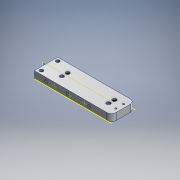
# Autodesk Inventor part: c-head-flange
Saved by Autodesk Inventor 2016 (Build 200138000, 138)
## iProperties
Created: 2015-05-12
Part Number: c-head-flange
Material: Aluminum 6061
Document SubType Name: Modeling
Designer: as
Mass: 12.4418 g
Surface Area: 45.4358 cm^2
Volume: 4.60808 cm^3
Density: 2.7 g/cm^3
Appearance: Aluminum - Flat
Author: as
Autodesk Inventor part; units mm, degrees
ref_plane "YZ Plane" through (0, 0, 0) normal (1, 0, 0) x (0, 1, 0)
ref_plane "XZ Plane" through (0, 0, 0) normal (0, 1, 0) x (-1, 0, 0)
ref_plane "XY Plane" through (0, 0, 0) normal (0, 0, 1) x (1, 0, 0)
sketch "Sketch1" plane through (0, 0, 0) normal (0, 0, 1) x (1, 0, 0)
  line L0 (-6, -20) -> (60, -20)
  line L1 (60, -20) -> (60, 0)
  line L2 (60, 0) -> (-6, 0)
  line L3 (-6, 0) -> (-6, -20)
  point P0 (0, 0)
  dimension "d2" = 20
  dimension "d3" = 66
  dimension "d8" = 60
  dimension "d9" = 0
  constraints: 8 end point, 2 parallel, 1 horizontal, 1 perpendicular
  measures "d2" distance of L0.end L1.end
  measures "d3" distance of L1.end L2.end
  measures "d8" distance from line of point (0, 0) L1
  measures "d9" distance from line of point (0, 0) L2
extrude "Extrusion1" add sketch "Sketch1" along normal blind 6
sketch "Sketch5" plane through (0, 0, 6) normal (0, 0, 1) x (1, 0, 0)
  line L0 (-6, 0) -> (-6, -20) projected
  point P0 (0, 0)
  point P1 (-3, -3)
  point P2 (-3, -17)
  dimension "d48" = 3
  dimension "d50" = 17
  dimension "d51" = 3
  dimension "d53" = 3
  measures "d48" horizontal distance of L0.start point (-3, -3)
  measures "d50" vertical distance of L0.start point (-3, -17)
  measures "d51" distance from line of L0 point (-3, -3)
  measures "d53" distance from line of L0 point (-3, -17)
hole "Hole6" at (-3, -3, 6) at (-3, -17, 6) direction (0, 0, -1) diameter 3 end through all
sketch "Sketch7" plane through (0, 0, 0) normal (0, 0, -1) x (-1, 0, 0)
  line L0 (-60, 0) -> (0, 0) projected
  line L1 (6, 0) -> (6, -20) projected
  point P0 (-57, -6.75)
  point P1 (-57, -13.25)
  dimension "d68" = 6.75
  dimension "d69" = 63
  dimension "d70" = 6.5
  dimension "d71" = 63
  measures "d68" distance from line of L0 point (-57, -6.75)
  measures "d69" distance from line of L1 point (-57, -6.75)
  measures "d70" distance of point (-57, -13.25) point (-57, -6.75)
  measures "d71" distance from line of point (-57, -13.25) L1
hole "Hole9" at (57, -13.25, 0) at (57, -6.75, 0) direction (0, 0, 1) diameter 1.567 end through all thread size "M2x0.4" class "6H" standard "ISO Metric profile"
sketch "Sketch8" plane through (0, 0, 0) normal (0, 0, -1) x (-1, 0, 0)
  line L0 (-51.7988, -18) -> (-47.7988, -18)
  line L1 (-47.7988, -2) -> (-51.7988, -2)
  line L2 (-53.7988, -4) -> (-53.7988, -16)
  line L3 (-53.7988, -18) -> (-45.7988, -2) construction
  line L4 (-45.7988, -18) -> (-53.7988, -2) construction
  arc A0 (-53.7988, -16) -> (-51.7988, -18) centre (-51.7988, -16) ccw
  arc A1 (-47.7988, -18) -> (-45.9448, -16.75) centre (-47.7988, -16) ccw
  arc A2 (-45.9448, -3.25) -> (-47.7988, -2) centre (-47.7988, -4) ccw
  arc A3 (-51.7988, -2) -> (-53.7988, -4) centre (-51.7988, -4) ccw
  line L5 (-44.0907, -15.5) -> (-1.7988, -15.5)
  line L6 (-1.7988, -4.5) -> (-44.0907, -4.5)
  line L7 (0.2012, -6.5) -> (0.2012, -13.5)
  arc A4 (-1.7988, -15.5) -> (0.2012, -13.5) centre (-1.7988, -13.5) ccw
  arc A5 (0.2012, -6.5) -> (-1.7988, -4.5) centre (-1.7988, -6.5) ccw
  arc A6 (-44.0907, -15.5) -> (-45.9448, -16.75) centre (-44.0907, -17.5) ccw
  arc A7 (-45.9448, -3.25) -> (-44.0907, -4.5) centre (-44.0907, -2.5) ccw
  line L8 (-60, 0) -> (6, 0) projected
  line L9 (6, -20) -> (-60, -20) projected
  point P0 (-49.7988, -10)
  point P1 (-45.7988, -16)
  point P2 (-45.8623, -4.5)
  point P3 (-44.7988, -15.5)
  dimension "d124" = 16
  dimension "d125" = 8
  dimension "d126" = 2
  dimension "d149" = 2
  dimension "d150" = 2
  dimension "d165" = 10
  dimension "d166" = 4.5
  dimension "d167" = 4.5
  dimension "d168" = 66
  dimension "d169" = 10
  dimension "d170" = 2
  dimension "d171" = 2
  dimension "d172" = 54
  dimension "d173" = 5.7988
  dimension "d174" = 4
  dimension "d175" = 45
  constraints: 18 point on circle, 16 end point, 16 tangent, 8 centre point, 8 point on line, 5 equal radius, 4 parallel, 2 midpoint, 1 horizontal, 1 vertical
  measures "d124" distance of L4.end L3.start
  measures "d125" distance of L3.start L4.start
  measures "d126" radius of A0
  measures "d149" radius of A4
  measures "d150" radius of A6
  measures "d165" distance from line of L8 point (-49.799, -10)
  measures "d166" distance between parallel lines of L8 L6
  measures "d167" distance between parallel lines of L9 L5
  measures "d168" distance of L8.start L8.end
  measures "d169" distance from line of point (-49.799, -10) L9
  measures "d170" distance between parallel lines of L8 L1
  measures "d171" distance between parallel lines of L9 L0
  measures "d172" distance between parallel lines of L7 L2
  measures "d173" distance from line of L8.end L7
  measures "d174" distance from line of point (-45.799, -16) L9
  measures "d175" distance from line of point (-44.799, -15.5) L7
extrude "Extrusion2" cut sketch "Sketch8" against normal blind 4.75
ref_plane "Work Plane1" through (-6, -10, 0) normal (0, 1, 0) x (1, 0, 0)
sketch "Sketch6" plane through (-6, -20, 0) normal (0, -1, 0) x (1, 0, 0)
  point P0 (43, 3)
  point P1 (30, 3)
  point P2 (17, 3)
sketch "Sketch11" plane through (0, 0, 4.75) normal (0, 0, -1) x (-1, 0, 0)
  point P0 (-10, -12.5)
hole "Hole12" at (10, -12.5, 4.75) direction (0, 0, 1) diameter 3.2 depth 1.25
sketch "Sketch13" plane through (-5.75, -20, 0) normal (0, -1, 0) x (1, 0, 0)
  point P0 (46.75, 3)
  point P1 (28.25, 3)
  point P2 (9.75, 3)
sketch "Sketch14" plane through (0, 0, 4.75) normal (0, 0, -1) x (-1, 0, 0)
  point P0 (-50, -12.5)
hole "Hole18" at (50, -12.5, 4.75) direction (0, 0, 1) diameter 3.4 depth 1.25
sketch "Sketch4" plane through (-6, -20, 0) normal (0, -1, 0) x (1, 0, 0)
  line L0 (6, 0) -> (66, 0) projected
  line L1 (0, 0) -> (0, 6) projected
  point P0 (10, 3)
  point P1 (28.5, 3)
  point P2 (47, 3)
  dimension "d42" = 4
  dimension "d43" = 22.5
  dimension "d44" = 41
  dimension "d45" = 3
  dimension "d46" = 3
  dimension "d47" = 3
  dimension "d146" = 6
  measures "d42" horizontal distance of L0.start point (10, 3)
  measures "d43" horizontal distance of point (28.5, 3) L0.start
  measures "d44" horizontal distance of L0.start point (47, 3)
  measures "d45" vertical distance of point (10, 3) L0.start
  measures "d46" distance from line of L0 point (28.5, 3)
  measures "d47" distance from line of L0 point (47, 3)
  measures "d146" distance from line of L1 L0.start
hole "Hole5" at (41, -20, 3) at (22.5, -20, 3) at (4, -20, 3) direction (0, 1, 0) diameter 2.459 end through all thread size "M3x0.5" class "6H" standard "ISO Metric profile"
mirror "Mirror3" about plane through (-6, -10, 0) normal (0, 1, 0) of "Hole12", "Hole18"
fillet "Fillet3" radius 4 2 edges at (60, -20, 3) (60, 0, 3)
equation "\"d3\" = d0"
equation "\"d53\" = d51"
equation "\"d165\" = 0.5 * d2"
equation "\"d167\" = d166"
equation "\"d43\" = 0.5 * d44 + 0.5 * d42"
equation "\"d46\" = d45"
equation "\"d47\" = d45"
equation "\"d36\" = d2"
equation "\"d0\" = 66"
body "Solid1"
